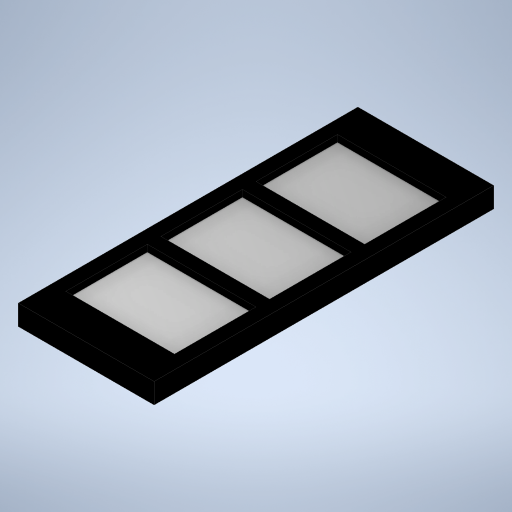
# Autodesk Inventor part: LED
Saved by Autodesk Inventor 2024 (Build 280153000, 153)
## iProperties
Created: 2024-06-13
Part Number: LED
Material: PC/ABS Plastic
Document SubType Name: Modeling
Designer: ASUS
Density: 0.357273 g/cm^3
Appearance: Anodized - Black
Author: ASUS
Autodesk Inventor part; units mm, degrees
ref_plane "YZ Plane" through (0, 0, 0) normal (1, 0, 0) x (0, 1, 0)
ref_plane "XZ Plane" through (0, 0, 0) normal (0, 1, 0) x (-1, 0, 0)
ref_plane "XY Plane" through (0, 0, 0) normal (0, 0, 1) x (1, 0, 0)
sketch "Sketch1" plane through (0, 0, 0) normal (0, 1, 0) x (-1, 0, 0)
  line L0 (0, 0) -> (20, 0)
  line L1 (20, 0) -> (20, -50)
  line L2 (20, -50) -> (0, -50)
  line L3 (0, -50) -> (0, 0)
  dimension "d0" = 20
  dimension "d1" = 50
  constraints: 8 end point, 2 parallel, 1 horizontal, 1 perpendicular
  measures "d0" distance between parallel lines of L3 L1
  measures "d1" distance between parallel lines of L2 L0
extrude "Extrusion1" add sketch "Sketch1" along normal blind 3
sketch "Sketch3" plane through (0, 3, 0) normal (0, 1, 0) x (1, 0, 0)
  line L0 (-18, 45) -> (-2, 45)
  line L1 (-2, 45) -> (-2, 33)
  line L2 (-2, 33) -> (-18, 33)
  line L3 (-18, 33) -> (-18, 45)
  line L4 (-18, 31) -> (-2, 31)
  line L5 (-2, 31) -> (-2, 19)
  line L6 (-2, 19) -> (-18, 19)
  line L7 (-18, 19) -> (-18, 31)
  line L8 (-18, 17) -> (-2, 17)
  line L9 (-2, 17) -> (-2, 5)
  line L10 (-2, 5) -> (-18, 5)
  line L11 (-18, 5) -> (-18, 17)
  line L12 (-20, 50) -> (-20, 0) projected
  line L13 (0, 0) -> (0, 50) projected
  line L14 (0, 50) -> (-20, 50) projected
  line L15 (-20, 0) -> (0, 0) projected
  point P0 (-18, 39)
  point P1 (-2, 39)
  point P2 (-10, 33)
  dimension "d14" = 2
  dimension "d15" = 2
  dimension "d16" = 5
  dimension "d17" = 5
  dimension "d22" = 12
  dimension "d23" = 12
  dimension "d24" = 12
  dimension "d25" = 2
  constraints: 24 end point, 6 parallel, 4 point on line, 3 horizontal, 3 midpoint, 3 perpendicular
  measures "d14" distance from line of L12 point (-18, 39)
  measures "d15" distance from line of L13 point (-2, 39)
  measures "d16" distance between parallel lines of L14 L0
  measures "d17" distance between parallel lines of L15 L10
  measures "d22" distance between parallel lines of L2 L0
  measures "d23" distance between parallel lines of L6 L4
  measures "d24" distance between parallel lines of L10 L8
  measures "d25" distance between parallel lines of L4 L2
extrude "Extrusion3" cut sketch "Sketch3" against normal blind 1 contours L0 L1 L2 L3 | L4 L5 L6 L7 | L8 L9 L10 L11
body "Solid1"
